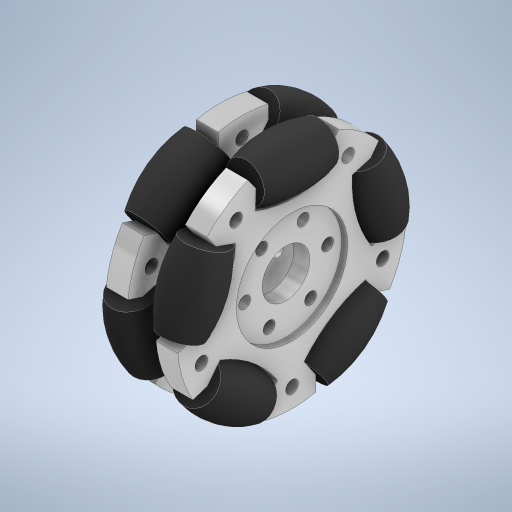
# Autodesk Inventor part: omni-60
Saved by Autodesk Inventor 2024.1 (Build 281209000, 209)
## iProperties
Created: 2024-02-10
Part Number: omni-60
Material: アルミニウム 6061
Document SubType Name: Modeling
Designer: haruy
Density: 2.7 g/cm^3
Appearance: アルミニウム - フラット
Author: haruy
Autodesk Inventor part; units mm, degrees
ref_plane "XZ Plane" through (0, 0, 0) normal (0, 1, 0) x (-1, 0, 0)
ref_plane "XY Plane" through (0, 0, 0) normal (0, 0, 1) x (1, 0, 0)
sketch "スケッチ1" plane through (0, 0, 0) normal (1, 0, 0) x (0, 1, 0)
  circle A0 centre (0, 0) radius 6
  circle A1 centre (0, 0) radius 10.5
  circle A2 centre (10.5, 0) radius 1.5
  circle A3 centre (5.25, 9.0933) radius 1.5
  circle A4 centre (-5.25, 9.0933) radius 1.5
  circle A5 centre (-10.5, 0) radius 1.5
  circle A6 centre (-5.25, -9.0933) radius 1.5
  circle A7 centre (5.25, -9.0933) radius 1.5
  circle A8 centre (0, 0) radius 24
  circle A9 centre (24, 0) radius 1.6
  circle A10 centre (7.4164, 22.8254) radius 1.6
  circle A11 centre (-19.4164, 14.1068) radius 1.6
  circle A12 centre (-19.4164, -14.1068) radius 1.6
  circle A13 centre (7.4164, -22.8254) radius 1.6
  circle A14 centre (0, 0) radius 14
  circle A15 centre (0, 0) radius 30 construction
  line L0 (19.3213, 24.952) -> (29.7114, 9.6453)
  line L1 (29.7114, 9.6453) -> (18.9554, 2.3441)
  line L2 (18.9554, 2.3441) -> (8.5652, 17.6508)
  line L3 (8.5652, 17.6508) -> (19.3213, 24.952)
  line L4 (13.7603, 9.9975) -> (24.5164, 17.2987)
  line L5 (13.9432, 21.3014) -> (24.3334, 5.9947)
  arc A16 (24.5123, 17.2958) -> (17.9614, 24.0289) centre (0, 0) ccw
  circle A17 centre (38.8872, 26.3967) radius 30 construction
  arc A18 (9.9251, 18.5739) -> (13.7644, 10.0001) centre (38.8872, 26.3967) ccw
  arc A19 (28.6432, 8.9202) -> (24.5123, 17.2958) centre (0, 0) ccw
  circle A20 centre (38.8872, 26.3967) radius 30 construction
  arc A21 (13.7644, 10.0001) -> (20.0237, 3.0693) centre (38.8872, 26.3967) ccw
  arc A22 (-14.5978, 15.179) -> (-5.2573, 16.181) centre (-13.0879, 45.141) ccw
  arc A23 (-5.2573, 16.181) -> (3.2686, 19.9921) centre (-13.0879, 45.141) ccw
  line L6 (-15.9501, 19.8433) -> (1.8181, 24.9949)
  line L7 (-14.1401, 13.6004) -> (-17.7602, 26.0862)
  line L8 (0.0081, 31.2378) -> (3.6282, 18.752)
  circle A24 centre (0, 0) radius 30 construction
  arc A25 (0.3676, 29.9977) -> (-8.8746, 28.6573) centre (0, 0) ccw
  arc A26 (-8.8746, 28.6573) -> (-17.3025, 24.5076) centre (0, 0) ccw
  arc A27 (-18.947, -9.1928) -> (-17.0136, 0.0002) centre (-46.976, 1.502) ccw
  arc A28 (-17.0136, 0.0002) -> (-18.0036, 9.2865) centre (-46.976, 1.502) ccw
  line L9 (-23.801, -9.0376) -> (-23.2098, 9.453)
  line L10 (-17.3043, -9.2453) -> (-30.2977, -8.8298)
  line L11 (-29.7064, 9.6607) -> (-16.7131, 9.2453)
  circle A29 centre (0, 0) radius 30 construction
  arc A30 (-28.4159, 9.6195) -> (-29.9971, 0.4154) centre (0, 0) ccw
  arc A31 (-29.9971, 0.4154) -> (-28.6549, -8.8824) centre (0, 0) ccw
  arc A32 (2.8879, -20.8604) -> (-5.2577, -16.1808) centre (-15.9449, -44.2127) ccw
  arc A33 (-5.2577, -16.1808) -> (-14.3954, -14.2527) centre (-15.9449, -44.2127) ccw
  line L12 (1.2403, -25.4288) -> (-16.1625, -19.1527)
  line L13 (3.4455, -19.3143) -> (-0.9648, -31.5433)
  line L14 (-18.3677, -25.2672) -> (-13.9574, -13.0381)
  circle A34 centre (0, 0) radius 30 construction
  arc A35 (-17.9297, -24.0526) -> (-9.6647, -28.4006) centre (0, 0) ccw
  arc A36 (-9.6647, -28.4006) -> (-0.4072, -29.9972) centre (0, 0) ccw
  arc A37 (20.7318, -3.6997) -> (13.7642, -10.0005) centre (37.1215, -28.8269) ccw
  arc A38 (13.7642, -10.0005) -> (9.1067, -18.0952) centre (37.1215, -28.8269) ccw
  line L15 (24.5675, -6.6783) -> (13.2208, -21.29)
  line L16 (19.4337, -2.6916) -> (29.7014, -10.665)
  line L17 (18.3546, -25.2767) -> (8.0869, -17.3033)
  circle A39 centre (0, 0) radius 30 construction
  arc A40 (17.3348, -24.4848) -> (24.024, -17.9679) centre (0, 0) ccw
  arc A41 (24.024, -17.9679) -> (28.4032, -9.657) centre (0, 0) ccw
  line L18 (-17.7602, 26.0862) -> (0.0081, 31.2378)
  line L19 (-30.2977, -8.8298) -> (-29.7064, 9.6607)
  line L20 (-0.9648, -31.5433) -> (-18.3677, -25.2672)
  line L21 (29.7014, -10.665) -> (18.3546, -25.2767)
  circle A42 centre (0, 0) radius 17
  circle A43 centre (0, 0) radius 28.8144
  line L22 (24.3334, 5.9947) -> (28.1839, 5.9947)
  line L23 (24.5675, -6.6783) -> (28.0298, -6.6783)
  line L24 (1.8181, 24.9949) -> (3.008, 28.657)
  line L25 (13.9432, 21.3014) -> (15.0132, 24.5942)
  line L26 (-23.2098, 9.453) -> (-26.3249, 11.7163)
  line L27 (-15.9501, 19.8433) -> (-18.7512, 21.8784)
  line L28 (-16.1625, -19.1527) -> (-19.2777, -21.4159)
  line L29 (-23.801, -9.0376) -> (-26.602, -11.0726)
  line L30 (13.2208, -21.29) -> (14.4106, -24.952)
  line L31 (1.2403, -25.4288) -> (2.3102, -28.7217)
  point P0 (-8.876, 28.662)
  point P1 (-30.002, 0.4154)
  point P2 (-9.6663, -28.4053)
  point P3 (24.028, -17.9709)
  point P4 (20.0237, 3.0693)
  point P5 (14.0656, 9.5477)
  point P6 (13.7644, 10.0002)
  point P7 (1.8181, 24.9949)
  point P8 (3.2686, 19.9921)
  point P9 (-14.5978, 15.179)
  point P10 (-23.2098, 9.453)
  point P11 (-18.0036, 9.2865)
  point P12 (-18.947, -9.1928)
  point P13 (-14.3954, -14.2527)
  point P14 (2.8879, -20.8604)
  point P15 (9.1067, -18.0952)
  point P16 (20.7318, -3.6997)
  dimension "d1" = 21
  dimension "d7" = 48
  dimension "d0" = 12
  dimension "d2" = 3
  dimension "d5" = 360
  dimension "d8" = 3.2
  dimension "d11" = 360
  dimension "d13" = 28
  dimension "d14" = 60
  dimension "d15" = 13
  dimension "d16" = 18.5
  dimension "d17" = 36
  dimension "d20" = 360
  dimension "d24" = 360
  dimension "d26" = 34
  dimension "d29" = 360
  constraints: 64 end point, 52 point on circle, 40 centre point, 18 coincident, 10 point on line, 7 symmetric about line, 4 midpoint, 2 horizontal, 2 horizontal alignment, 2 parallel, 1 perpendicular, 1 tangent, 216 other
  measures "d0" diameter of A0
  measures "d2" diameter of A2
  measures "d8" diameter of A9
  measures "d13" diameter of A14
  measures "d14" diameter of A15
  measures "d15" distance of L0.end L1.end
  measures "d16" distance of L0.start L0.end
  measures "d26" diameter of A42
extrude "押し出し1" add sketch "スケッチ1" along normal mid plane 5.5 contours A2 A1 A7 A6 A5 A4 A3 | A9 A8 L16 A37 A38 A42 L2 L1 | A8 L1 L22 A43 L23 L16 A9 | L1 L2 A21 | A42 A23 L8 A8 A10 L3 L2 | A42 | L4 L2 L3 A18 | A42 A28 L11 A8 A11 L7 A22 A23 | L17 L30 A43 L31 L13 A8 A13 | A8 A13 L13 A32 A33 A42 A38 L17 | A8 A10 L8 L24 A43 L25 L3 | A42 A33 L14 A8 A12 L10 A27 A28 | A8 A11 L11 L26 A43 L27 L7 | L14 L28 A43 L29 L10 A8 A12 | A14
revolve "回転1" add sketch "スケッチ1" angle 360 about axis through (0, 13.9432, 21.3014) along (0, 0.5616311, -0.8273877) separate body contours L5 L4 A8 | A8 L4 A43 L1 L5 | L4 L5 A8 | A8 L5 L3 A43 L4 | A43 L4 A19 L1 | A43 L3 A16 L4
pattern_circular "円形状パターン1" count 5 over 360 about axis through (-10, 0, 0) along (1, 0, 0) of "回転1" bodies 2
ref_plane "作業平面1" through (12.6, 0, 0) normal (1, 0, 0) x (0, 1, 0)
sketch "スケッチ3" plane through (12.6, 0, 0) normal (1, 0, 0) x (0, 1, 0)
  circle A0 centre (0, 0) radius 6
  circle A1 centre (0, 0) radius 10.5
  circle A2 centre (8.4947, 6.1717) radius 1.5
  circle A3 centre (-1.0975, 10.4425) radius 1.5
  circle A4 centre (-9.5922, 4.2707) radius 1.5
  circle A5 centre (-8.4947, -6.1717) radius 1.5
  circle A6 centre (1.0975, -10.4425) radius 1.5
  circle A7 centre (9.5922, -4.2707) radius 1.5
  circle A8 centre (0, 0) radius 24
  circle A9 centre (19.4164, 14.1068) radius 1.6
  circle A10 centre (-7.4164, 22.8254) radius 1.6
  circle A11 centre (-24, 0) radius 1.6
  circle A12 centre (-7.4164, -22.8254) radius 1.6
  circle A13 centre (19.4164, -14.1068) radius 1.6
  circle A14 centre (0, 0) radius 14
  circle A15 centre (0, 0) radius 30 construction
  line L0 (0.9648, 31.5433) -> (18.3677, 25.2672)
  line L1 (18.3677, 25.2672) -> (13.9574, 13.0381)
  line L2 (13.9574, 13.0381) -> (-3.4455, 19.3143)
  line L3 (-3.4455, 19.3143) -> (0.9648, 31.5433)
  line L4 (5.256, 16.1762) -> (9.6663, 28.4053)
  line L5 (-1.2403, 25.4288) -> (16.1625, 19.1527)
  arc A16 (9.6647, 28.4006) -> (0.4072, 29.9972) centre (0, 0) ccw
  circle A17 centre (15.9449, 44.2127) radius 30 construction
  arc A18 (-2.8879, 20.8604) -> (5.2577, 16.1808) centre (15.9449, 44.2127) ccw
  arc A19 (17.9297, 24.0526) -> (9.6647, 28.4006) centre (0, 0) ccw
  circle A20 centre (15.9449, 44.2127) radius 30 construction
  arc A21 (5.2577, 16.1808) -> (14.3954, 14.2527) centre (15.9449, 44.2127) ccw
  arc A22 (-20.7318, 3.6997) -> (-13.7642, 10.0005) centre (-37.1215, 28.8269) ccw
  arc A23 (-13.7642, 10.0005) -> (-9.1067, 18.0952) centre (-37.1215, 28.8269) ccw
  line L6 (-24.5675, 6.6783) -> (-13.2208, 21.29)
  line L7 (-19.4337, 2.6916) -> (-29.7014, 10.665)
  line L8 (-18.3546, 25.2767) -> (-8.0869, 17.3033)
  circle A24 centre (0, 0) radius 30 construction
  arc A25 (-17.3348, 24.4848) -> (-24.024, 17.9679) centre (0, 0) ccw
  arc A26 (-24.024, 17.9679) -> (-28.4032, 9.657) centre (0, 0) ccw
  arc A27 (-9.9251, -18.5739) -> (-13.7644, -10.0001) centre (-38.8872, -26.3967) ccw
  arc A28 (-13.7644, -10.0001) -> (-20.0237, -3.0693) centre (-38.8872, -26.3967) ccw
  line L9 (-13.9432, -21.3014) -> (-24.3334, -5.9947)
  line L10 (-8.5652, -17.6508) -> (-19.3213, -24.952)
  line L11 (-29.7114, -9.6453) -> (-18.9554, -2.3441)
  circle A29 centre (0, 0) radius 30 construction
  arc A30 (-28.6432, -8.9202) -> (-24.5123, -17.2958) centre (0, 0) ccw
  arc A31 (-24.5123, -17.2958) -> (-17.9614, -24.0289) centre (0, 0) ccw
  arc A32 (14.5978, -15.179) -> (5.2573, -16.181) centre (13.0879, -45.141) ccw
  arc A33 (5.2573, -16.181) -> (-3.2686, -19.9921) centre (13.0879, -45.141) ccw
  line L12 (15.9501, -19.8433) -> (-1.8181, -24.9949)
  line L13 (14.1401, -13.6004) -> (17.7602, -26.0862)
  line L14 (-0.0081, -31.2378) -> (-3.6282, -18.752)
  circle A34 centre (0, 0) radius 30 construction
  arc A35 (-0.3676, -29.9977) -> (8.8746, -28.6573) centre (0, 0) ccw
  arc A36 (8.8746, -28.6573) -> (17.3025, -24.5076) centre (0, 0) ccw
  arc A37 (18.947, 9.1928) -> (17.0136, -0.0002) centre (46.976, -1.502) ccw
  arc A38 (17.0136, -0.0002) -> (18.0036, -9.2865) centre (46.976, -1.502) ccw
  line L15 (23.801, 9.0376) -> (23.2098, -9.453)
  line L16 (17.3043, 9.2453) -> (30.2977, 8.8298)
  line L17 (29.7064, -9.6607) -> (16.7131, -9.2453)
  circle A39 centre (0, 0) radius 30 construction
  arc A40 (28.4159, -9.6195) -> (29.9971, -0.4154) centre (0, 0) ccw
  arc A41 (29.9971, -0.4154) -> (28.6549, 8.8824) centre (0, 0) ccw
  line L18 (-29.7014, 10.665) -> (-18.3546, 25.2767)
  line L19 (-19.3213, -24.952) -> (-29.7114, -9.6453)
  line L20 (17.7602, -26.0862) -> (-0.0081, -31.2378)
  line L21 (30.2977, 8.8298) -> (29.7064, -9.6607)
  circle A42 centre (0, 0) radius 17
  circle A43 centre (0, 0) radius 28.8144
  line L22 (16.1625, 19.1527) -> (19.2777, 21.4159)
  line L23 (23.801, 9.0376) -> (26.602, 11.0726)
  line L24 (-13.2208, 21.29) -> (-14.4106, 24.952)
  line L25 (-1.2403, 25.4288) -> (-2.3102, 28.7217)
  line L26 (-24.3334, -5.9947) -> (-28.1839, -5.9947)
  line L27 (-24.5675, 6.6783) -> (-28.0298, 6.6783)
  line L28 (-1.8181, -24.9949) -> (-3.008, -28.657)
  line L29 (-13.9432, -21.3014) -> (-15.0132, -24.5942)
  line L30 (23.2098, -9.453) -> (26.3249, -11.7163)
  line L31 (15.9501, -19.8433) -> (18.7512, -21.8784)
  point P0 (-24.028, 17.9709)
  point P1 (-24.5164, -17.2987)
  point P2 (8.876, -28.662)
  point P3 (30.002, -0.4154)
  point P4 (21.2728, -7.1251)
  point P5 (15.3147, -0.6467)
  point P6 (15.0135, -0.1942)
  point P7 (11.1742, 8.3795)
  point P8 (15.1923, 11.107)
  point P9 (16.2623, 14.3998)
  point P10 (4.2571, 18.4626)
  point P11 (3.0672, 14.8005)
  point P12 (4.5177, 9.7977)
  point P13 (-13.3487, 4.9846)
  point P14 (-14.701, 9.6489)
  point P15 (-17.5021, 11.684)
  point P16 (-25.0758, 1.5219)
  point P17 (-21.9607, -0.7414)
  point P18 (-16.7545, -0.9079)
  point P19 (-17.6979, -19.3872)
  point P20 (-22.5519, -19.232)
  point P21 (-25.3529, -21.267)
  point P22 (-18.0286, -31.6103)
  point P23 (-14.9134, -29.3471)
  point P24 (-13.1463, -24.4471)
  point P25 (4.137, -31.0548)
  point P26 (2.4894, -35.6232)
  point P27 (3.5593, -38.9161)
  point P28 (15.6597, -35.1465)
  point P29 (14.4699, -31.4844)
  point P30 (10.3558, -28.2896)
  point P31 (21.9809, -13.8941)
  point P32 (14.3954, 14.2527)
  point P33 (5.7673, 15.9918)
  point P34 (5.2576, 16.1809)
  point P35 (-2.8879, 20.8604)
  point P36 (-9.1067, 18.0952)
  point P37 (-20.7318, 3.6997)
  point P38 (-20.0237, -3.0693)
  point P39 (-9.9251, -18.5739)
  point P40 (-1.8181, -24.9949)
  point P41 (-3.2686, -19.9921)
  point P42 (14.5978, -15.179)
  point P43 (23.2098, -9.453)
  point P44 (18.0036, -9.2865)
  point P45 (18.947, 9.1928)
  dimension "d20" = 360
  dimension "d75" = 21
  dimension "d78" = 48
  dimension "d74" = 12
  dimension "d76" = 3
  dimension "d77" = 360
  dimension "d79" = 3.2
  dimension "d80" = 360
  dimension "d81" = 28
  dimension "d82" = 60
  dimension "d83" = 13
  dimension "d84" = 18.5
  dimension "d85" = 36
  dimension "d86" = 360
  dimension "d87" = 360
  dimension "d88" = 34
  dimension "d89" = 360
  dimension "d90" = 0
  dimension "d91" = 0
  constraints: 64 end point, 52 point on circle, 42 centre point, 18 coincident, 10 point on line, 7 symmetric about line, 4 midpoint, 2 parallel, 1 perpendicular, 1 tangent, 210 other
  measures "d74" diameter of A0
  measures "d76" diameter of A2
  measures "d79" diameter of A9
  measures "d81" diameter of A14
  measures "d82" diameter of A15
  measures "d83" distance of L0.end L1.end
  measures "d84" distance of L0.start L0.end
  measures "d88" diameter of A42
  measures "d90" distance of point (0, 0) point (0, 0)
  measures "d91" distance of point (0, 0) point (0, 0)
extrude "押し出し2" add sketch "スケッチ3" along normal mid plane 5.5 separate body contours A1 A7 A6 A5 A4 A3 A2 | L16 A37 A38 A42 L2 L1 A8 A9 | A8 A9 L1 L22 A43 L23 L16 | L17 L30 A43 L31 L13 A8 A13 | A8 A13 L13 A32 A33 A42 A38 L17 | A42 | A33 L14 A8 A12 L10 A27 A28 A42 | L1 L2 A21 | A28 L11 A8 A11 L7 A22 A23 A42 | A42 A23 L8 A8 A10 L3 L2 | L14 L28 A43 L29 L10 A8 A12 | L2 L3 A18 L4 | L3 A8 A10 L8 L24 A43 L25 | L11 L26 A43 L27 L7 A8 A11 | A14
revolve "回転2" add sketch "スケッチ3" angle 360 about axis through (12.6, -1.2403, 25.4288) along (0, 0.9406954, -0.3392522) separate body contours A43 L4 A19 L1 | L1 L5 A8 L4 A43 | L5 L4 A8 | A43 L3 A16 L4 | L4 A8 L5 L3 A43 | L4 L5 A8
pattern_circular "円形状パターン2" count 5 over 360 about axis through (-10, 0, 0) along (1, 0, 0) of "回転2" bodies 4
sketch "スケッチ4" plane through (15.35, 0, 0) normal (1, 0, 0) x (0, 0, -1)
  circle A0 centre (0, 0) radius 14
  circle A1 centre (10.4425, 1.0975) radius 1.5 projected
  circle A2 centre (10.4425, 1.0975) radius 1.5
  circle A3 centre (4.2707, 9.5922) radius 1.5
  circle A4 centre (-6.1717, 8.4947) radius 1.5
  circle A5 centre (-10.4425, -1.0975) radius 1.5
  circle A6 centre (-4.2707, -9.5922) radius 1.5
  circle A7 centre (6.1717, -8.4947) radius 1.5
  dimension "d98" = 28
  dimension "d101" = 360
  constraints: 7 centre point, 2 coincident, 13 other
  measures "d98" diameter of A0
extrude "押し出し3" cut sketch "スケッチ4" against normal blind 1.5 bodies 3
sketch "スケッチ5" plane through (-2.75, 0, 0) normal (-1, 0, 0) x (0, 0, 1)
  circle A0 centre (0, 0) radius 14
  circle A1 centre (0, 10.5) radius 1.5 projected
  circle A2 centre (0, 10.5) radius 1.5
  circle A3 centre (-9.0933, 5.25) radius 1.5
  circle A4 centre (-9.0933, -5.25) radius 1.5
  circle A5 centre (0, -10.5) radius 1.5
  circle A6 centre (9.0933, -5.25) radius 1.5
  circle A7 centre (9.0933, 5.25) radius 1.5
  dimension "d105" = 28
  dimension "d108" = 360
  constraints: 7 centre point, 2 coincident, 13 other
  measures "d105" diameter of A0
extrude "押し出し4" cut sketch "スケッチ5" against normal blind 1.5 bodies 1
